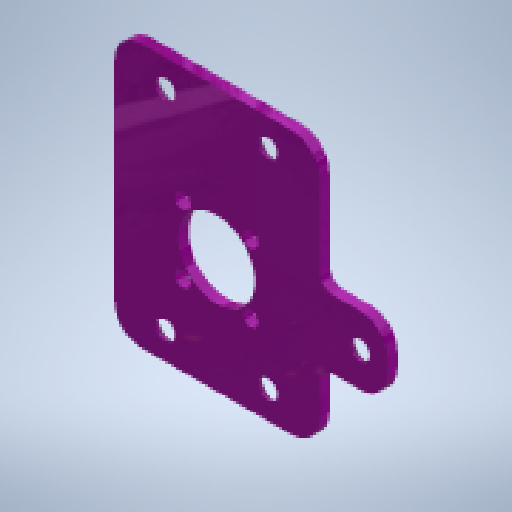
# Autodesk Inventor part: кронштейн
Saved by Autodesk Inventor 2025 (Build 290162000, 162)
## iProperties
Created: 2025-02-17
Part Number: кронштейн
Material: Сталь
Document SubType Name: Sheet Metal
Designer: volko
Density: 7.85 g/cm^3
Sheet Metal Rule: По умолчанию_мм
Appearance: Гладкий — пурпурный
Mass: 145.221 g
Surface Area: 142.245 cm^2
Volume: 18.4995 cm^3
Author: volko
Autodesk Inventor part; units mm, degrees
ref_plane "YZ Plane" through (0, 0, 0) normal (1, 0, 0) x (0, 1, 0)
ref_plane "XZ Plane" through (0, 0, 0) normal (0, 1, 0) x (-1, 0, 0)
ref_plane "XY Plane" through (0, 0, 0) normal (0, 0, 1) x (1, 0, 0)
sketch "Эскиз1" plane through (0, 0, 0) normal (0, 0, 1) x (1, 0, 0)
  line L0 (-1.5933, 45.7) -> (22, 45.7)
  line L1 (30, 37.7) -> (30, 10)
  arc A0 (30, 37.7) -> (22, 45.7) centre (22, 37.7) ccw
  line L2 (-1.5933, 45.7) -> (-22, 45.7)
  line L3 (-30, 37.7) -> (-30, -6.25)
  arc A1 (-22, 45.7) -> (-30, 37.7) centre (-22, 37.7) ccw
  line L4 (30, -20.5) -> (30, -10)
  line L5 (-30, -20.5) -> (-30, -6.25)
  line L6 (-48.3196, 0) -> (68.3196, 0) projected
  line L7 (0, -45.6596) -> (0, 62.8596) projected
  circle A2 centre (0, 2) radius 11.25
  circle A3 centre (0, 2) radius 14 construction
  line L8 (0, 2) -> (-9.8995, 11.8995) construction
  line L9 (-22, -28.5) -> (22, -28.5)
  arc A4 (-30, -20.5) -> (-22, -28.5) centre (-22, -20.5) ccw
  arc A5 (22, -28.5) -> (30, -20.5) centre (22, -20.5) ccw
  line L10 (30, -10) -> (42, -10)
  line L11 (50, -2) -> (50, 2)
  line L12 (42, 10) -> (30, 10)
  arc A6 (50, 2) -> (42, 10) centre (42, 2) ccw
  arc A7 (42, -10) -> (50, -2) centre (42, -2) ccw
  point P0 (0, 0)
  point P1 (0, 0)
  point P2 (30, -28.5)
  point P3 (-30, -28.5)
  point P4 (15, 37.7)
  point P5 (-15, 37.7)
  point P6 (9.8995, 11.8995)
  point P7 (-9.8995, -7.8995)
  point P8 (9.8995, -7.8995)
  point P9 (15, -20.5)
  point P10 (-15, -20.5)
  point P11 (42, 0)
  dimension "d128" = 28
  dimension "d4" = 60
  dimension "d43" = 8
  dimension "d50" = 30
  dimension "d127" = 22.5
  dimension "d131" = 360
  dimension "d134" = 45
  dimension "d168" = 8
  dimension "d182" = 2
  dimension "d184" = 37.7
  dimension "d187" = 30
  dimension "d192" = 20.5
  dimension "d193" = 8
  dimension "d196" = 20
  dimension "d197" = 20
  dimension "d199" = 8
  constraints: 22 end point, 12 point on circle, 12 tangent, 7 centre point, 5 equal radius, 5 point on line, 4 horizontal, 3 perpendicular, 2 horizontal alignment, 2 vertical, 1 coincident, 1 collinear, 1 parallel, 12 other
  measures "d4" distance between parallel lines of L1 L3
  measures "d43" radius of A0
  measures "d50" distance of point (15, 37.7) point (-15, 37.7)
  measures "d127" diameter of A2
  measures "d134" angle of L8 L6
  measures "d168" distance from line of L0 point (15, 37.7)
  measures "d182" distance from line of L6 L8.start
  measures "d184" distance from line of L6 point (15, 37.7)
  measures "d187" distance of point (15, -20.5) point (-15, -20.5)
  measures "d192" distance from line of point (15, -20.5) L6
  measures "d193" distance from line of point (15, -20.5) L9
  measures "d196" distance between parallel lines of L10 L12
  measures "d197" distance between parallel lines of L1 L11
  measures "d199" distance from line of point (42, 0) L11
extrude "Пластина2" add sketch "Эскиз1" along normal blind 3 contours L0 L7 A2 L6 L3 A1 L2 | L0 A0 L1 L12 A6 L11 L6 A2 L7 | A2 L7 L9 A4 L5 L3 L6 | L6 L11 A7 L10 L4 A5 L9 L7 A2
hole "Отверстие2" at (-15, 37.7, 0) at (15, 37.7, 0) at (15, -20.5, 0) at (-15, -20.5, 0) at (42, 0, 0) direction (0, 0, 1) diameter 5.5 end through all countersink diameter 10.5 countersink angle 90
sketch "Эскиз6" plane through (0, 0, 3) normal (0, 0, 1) x (1, 0, 0)
  circle A0 centre (0, 2) radius 14 construction
  line L0 (0, -45.6596) -> (0, 62.8596) projected
  line L1 (-48.3196, 0) -> (68.3196, 0) projected
  line L2 (0, 2) -> (9.8995, 11.8995) construction
  point P0 (-9.8995, 11.8995)
  point P1 (-9.8995, -7.8995)
  point P2 (9.8995, -7.8995)
  dimension "d135" = 28
  dimension "d138" = 360
  dimension "d141" = 135
  dimension "d183" = 2
  constraints: 2 end point, 1 point on line, 8 other
  measures "d141" angle of L2 L1
  measures "d183" distance from line of L1 L2.start
hole "Отверстие3" at (-9.8995, -7.8995, 3) at (9.8995, 11.8995, 3) at (-9.8995, 11.8995, 3) at (9.8995, -7.8995, 3) direction (0, 0, -1) diameter 4.5 end through all
fillet "Сопряжение1" radius 4 2 edges at (30, 10, 1.5) (30, -10, 1.5)
equation "\"d18\" = Толщина"
equation "\"Радиус_гибки\" = Толщина"
equation "\"Ширина_просечки\" = Толщина"
equation "\"Глубина_просечки\" = 0.5 * Толщина"
equation "\"Размер_просечки\" = 4 * Толщина"
equation "\"Мин_остаток\" = 2 * Толщина"
equation "\"Радиус_перехода\" = Радиус_гибки"
equation "\"Радиус_Якоби\" = Радиус_гибки"
equation "\"Размер_зазора\" = Толщина"
equation "\"Толщина\" = 3"
